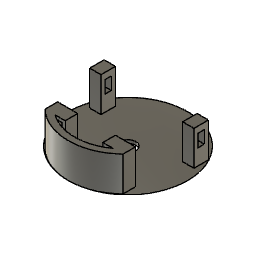
Socle dessus v3 (Autodesk Fusion 360 design; units mm, degrees)
Autodesk Fusion 360 part; units mm, degrees
sketch "Esquisse1" plane through (0, 0, 0) normal (0, 0, 1) x (1, 0, 0)
  circle A0 centre (0, 0) radius 95
  circle A1 centre (0, 0) radius 12.5
  dimension "d1" = 190
  dimension "d2" = 25
  constraint coincident A0.centre A1.centre
  measures "d1" diameter of A0
  measures "d2" diameter of A1
extrude "Extrusion1" add sketch "Esquisse1" along normal blind 5
sketch "Esquisse2" plane through (0, 0, 5) normal (0, 0, 1) x (-1, 0, 0)
  circle A0 centre (0, 0) radius 12.5
  circle A1 centre (0, 0) radius 95
  line L0 (30, 50) -> (30, 70)
  line L1 (-65, -45) -> (-83, -45)
  line L2 (30, 70) -> (62, 70)
  line L3 (-30, 70) -> (-62, 70)
  line L4 (0, -1.75) -> (0, -22.5)
  line L5 (-65, -22) -> (-65, -45)
  arc A2 (62, 70) -> (-62, 70) centre (0, 5.62) ccw
  circle A3 centre (0, 0) radius 17.5
  arc A4 (46, 70) -> (-46, 70) centre (0, 6.9667) ccw
  line L6 (65, -22) -> (65, -45)
  line L7 (65, -45) -> (83, -45)
  line L8 (1.75, 0) -> (22.5, 0)
  line L9 (-30, 50) -> (-30, 70)
  line L10 (-62, 70) -> (-62, 50)
  line L11 (-83, -22) -> (-65, -22)
  line L12 (62, 70) -> (62, 50)
  circle A5 centre (0, 0) radius 95
  line L13 (-83, -45) -> (-83, -22)
  line L14 (83, -45) -> (83, -22)
  line L15 (62, 50) -> (30, 50)
  line L16 (-62, 50) -> (-30, 50)
  line L17 (83, -22) -> (65, -22)
  dimension "d125" = 65
  dimension "d126" = 22
  dimension "d127" = 23
  dimension "d128" = 18
  dimension "d129" = 20
  dimension "d130" = 32
  dimension "d131" = 50
  dimension "d132" = 30
  constraint horizontal L11
  constraint vertical L5
  constraint horizontal L1
  constraint vertical L13
  constraint symmetric L11.start L14.end L4
  constraint symmetric L6.start L5.start L4
  constraint symmetric L6.end L1.start L4
  constraint symmetric L1.end L7.end L4
  constraint horizontal L16
  constraint vertical L9
  constraint horizontal L3
  constraint vertical L10
  constraint symmetric L10.end L12.end L4
  constraint symmetric L9.start L0.start L4
  constraint symmetric L3.start L0.end L4
  constraint symmetric L2.end L3.end L4
  constraint tangent A2 A5
  constraint midpoint A4.start L2
  constraint midpoint A4.end L3
  measures "d125" distance of L4 L5
  measures "d126" distance of L8 L11
  measures "d127" distance of L1 L11
  measures "d128" distance of L5 L13
  measures "d129" distance of L3 L16
  measures "d130" distance of L9 L10
  measures "d131" distance of L8 L16
  measures "d132" distance of L4 L9
extrude "Extrusion2" add sketch "Esquisse2" along normal blind 55 contours L2 L3 A2 A4 | L0 L2 L12 L15 | L3 L9 L10 L16 | L1 L5 L11 L13 | L6 L7 L14 L17
fillet "Congé1" radius 95 1 edges at (-88.5711, -34.3535, 0)
sketch "Esquisse3" plane through (83, 0, 0) normal (1, 0, 0) x (0, 1, 0)
  line L0 (22, 5) -> (45, 5)
  line L1 (45, 5) -> (45, 60)
  line L2 (45, 60) -> (22, 60)
  line L3 (22, 60) -> (22, 5)
  line L4 (28.5, 50) -> (38.5, 50)
  line L5 (38.5, 50) -> (38.5, 30)
  line L6 (38.5, 30) -> (28.5, 30)
  line L7 (28.5, 30) -> (28.5, 50)
  dimension "d17" = 10
  dimension "d18" = 6.5
  dimension "d19" = 20
  constraint horizontal L4
  constraint vertical L5
  constraint horizontal L6
  constraint vertical L7
  measures "d17" distance of L5 L7
  measures "d18" distance of L3 L7
  measures "d19" distance of L4 L6
extrude "Extrusion3" cut sketch "Esquisse3" against normal blind 30 contours L4 L5 L6 L7
sketch "Esquisse4" plane through (-65, 0, 0) normal (1, 0, 0) x (0, 1, 0)
  line L0 (22, 5) -> (45, 5)
  line L1 (45, 5) -> (45, 60)
  line L2 (45, 60) -> (22, 60)
  line L3 (22, 60) -> (22, 5)
  line L4 (28.5, 50) -> (38.5, 50)
  line L5 (38.5, 50) -> (38.5, 30)
  line L6 (38.5, 30) -> (28.5, 30)
  line L7 (28.5, 30) -> (28.5, 50)
  dimension "d22" = 10
  dimension "d23" = 6.5
  dimension "d24" = 20
  dimension "d25" = 10
  constraint horizontal L4
  constraint vertical L5
  constraint horizontal L6
  constraint vertical L7
  measures "d22" distance of L5 L7
  measures "d23" distance of L3 L7
  measures "d24" distance of L4 L6
  measures "d25" distance of L2 L4
extrude "Extrusion4" cut sketch "Esquisse4" against normal blind 40 contours L4 L5 L6 L7
sketch "Esquisse5" plane through (0, -50, 0) normal (0, 1, 0) x (-1, 0, 0)
  line L0 (-62, 5) -> (-30, 5)
  line L1 (-30, 5) -> (-30, 60)
  line L2 (-30, 60) -> (-62, 60)
  line L3 (-62, 60) -> (-62, 5)
  line L4 (-50, 55) -> (-35, 55)
  line L5 (-35, 55) -> (-35, 35)
  line L6 (-35, 35) -> (-50, 35)
  line L7 (-50, 35) -> (-50, 55)
  arc A0 through (46, 60, -20) (0, 60, -35) (-46, 60, -20)
  line L8 (35, 55) -> (50, 55)
  line L9 (50, 55) -> (50, 35)
  line L10 (50, 35) -> (35, 35)
  line L11 (35, 35) -> (35, 55)
  line L12 (30, 5) -> (30, 60)
  line L13 (30, 60) -> (62, 60)
  point P0 (-30, 5)
  point P1 (30, 5)
  dimension "d29" = 5
  dimension "d30" = 15
  dimension "d31" = 20
  dimension "d32" = 5
  dimension "d33" = 15
  dimension "d34" = 5
  dimension "d35" = 20
  dimension "d37" = 5
  constraint horizontal L4
  constraint vertical L5
  constraint horizontal L6
  constraint vertical L7
  constraint horizontal L8
  constraint vertical L9
  constraint horizontal L10
  constraint vertical L11
  measures "d29" distance of L2 L4
  measures "d30" distance of L5.end L6.end
  measures "d31" distance of L4.start L6.end
  measures "d32" distance of L1 L5
  measures "d33" distance of L8.start L8.end
  measures "d34" distance of L11 L12
  measures "d35" distance of L8.end L9.end
  measures "d37" distance of L8 L13
extrude "Extrusion5" cut sketch "Esquisse5" against normal blind 20 contours L4 L5 L6 L7 | L8 L9 L10 L11
